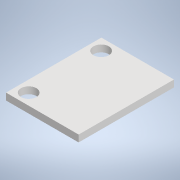
# Autodesk Inventor part: 10_MPU_6050
Saved by Autodesk Inventor 2020 (Build 240168000, 168)
## iProperties
Created: 2019-10-15
Part Number: 10_MPU_6050
Material: Generico
Document SubType Name: Modeling
Designer: socci
Density: 1 g/cm^3
Appearance: Default
Author: socci
Autodesk Inventor part; units mm, degrees
ref_plane "YZ Plane" through (0, 0, 0) normal (1, 0, 0) x (0, 1, 0)
ref_plane "XZ Plane" through (0, 0, 0) normal (0, 1, 0) x (-1, 0, 0)
ref_plane "XY Plane" through (0, 0, 0) normal (0, 0, 1) x (1, 0, 0)
sketch "Schizzo1" plane through (0, 0, 0) normal (0, 1, 0) x (-1, 0, 0)
  line L0 (10.5, 8) -> (-10.5, 8)
  line L1 (-10.5, 8) -> (-10.5, -8)
  line L2 (-10.5, -8) -> (10.5, -8)
  line L3 (10.5, -8) -> (10.5, 8)
  line L4 (10.5, 8) -> (-10.5, -8) construction
  line L5 (-10.5, 8) -> (10.5, -8) construction
  point P0 (0, 0)
  point P1 (0, 0)
  point P2 (0, 0)
  dimension "d0" = 16
  dimension "d1" = 21
  constraints: 12 end point, 3 midpoint, 2 parallel, 1 coincident, 1 horizontal, 1 perpendicular
  measures "d0" distance of L0.end L1.end
  measures "d1" distance of L0.start L0.end
extrude "Estrusione1" add sketch "Schizzo1" along normal blind 1.5
sketch "Schizzo2" plane through (0, 1.5, 0) normal (0, 1, 0) x (1, 0, 0)
  line L0 (10.5, 8) -> (-10.5, 8) projected
  line L1 (-10.5, 8) -> (-8, 8)
  line L2 (-8, 8) -> (-8, 5.5)
  line L3 (10.5, 8) -> (8, 8)
  line L4 (8, 8) -> (8, 5.5)
  point P0 (0, 0)
  dimension "d16" = 2.5
  dimension "d17" = 2.5
  dimension "d18" = 2.5
  dimension "d19" = 2.5
  constraints: 8 end point, 2 perpendicular, 2 point on line
  measures "d16" distance of L0.end L1.end
  measures "d17" distance of L1.end L2.end
  measures "d18" distance of L0.start L3.end
  measures "d19" distance of L3.end L4.end
hole "Foro1" at (-8, 1.5, -5.5) at (8, 1.5, -5.5) direction (0, -1, 0) diameter 3.4 depth 1.5 tip angle 118 clearance for "Vite a testa esagonale" size "M3" standard "ANSI - Profilo M Metrico"
